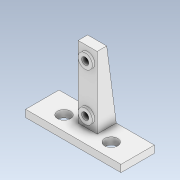
# Autodesk Inventor part: limit_switch_horizontal
Saved by Autodesk Inventor 2022 (Build 260153000, 153)
## iProperties
Created: 2022-05-08
Part Number: limit_switch_horizontal
Material: Generic
Document SubType Name: Modeling
Designer: ferna
Density: 1 g/cm^3
Appearance: White
Author: ferna
Autodesk Inventor part; units mm, degrees
ref_plane "YZ Plane" through (0, 0, 0) normal (1, 0, 0) x (0, 1, 0)
ref_plane "XZ Plane" through (0, 0, 0) normal (0, 1, 0) x (-1, 0, 0)
ref_plane "XY Plane" through (0, 0, 0) normal (0, 0, 1) x (1, 0, 0)
sketch "Sketch1" plane through (0, 0, 0) normal (0, 1, 0) x (-1, 0, 0)
  circle A0 centre (30.1, 6) radius 2.1
  circle A1 centre (49.9, 6) radius 2.1
  line L0 (0, 0) -> (80, 0)
  line L1 (80, 0) -> (80, 12)
  line L2 (0, 12) -> (80, 12)
  line L3 (0, 0) -> (0, 12)
  line L4 (40, 12) -> (15, 12)
  line L5 (15, 12) -> (15, 0)
  line L6 (15, 0) -> (65, 0)
  line L7 (65, 0) -> (65, 12)
  circle A2 centre (49.9, 6) radius 2.75
  circle A3 centre (30.1, 6) radius 2.75
  dimension "d0" = 25
  dimension "d1" = 50
  dimension "d2" = 5.5
  dimension "d3" = 5.5
  constraints: 16 end point, 4 centre point, 4 point on line, 2 coincident, 2 perpendicular, 1 midpoint
  measures "d0" distance of L4.start L4.end
  measures "d1" distance of L5.end L6.end
  measures "d2" diameter of A2
  measures "d3" diameter of A3
extrude "Extrusion1" add sketch "Sketch1" along normal blind 3 contours L5 L2 L7 L0
sketch "Sketch6" plane through (0, 3, 0) normal (0, 1, 0) x (1, 0, 0)
  line L0 (-15, 0) -> (-65, 0) projected
  line L1 (-40, 0) -> (-43, 0)
  line L2 (-65, -12) -> (-15, -12) projected
  line L3 (-40, -12) -> (-40, -8)
  line L4 (-40, -8) -> (-43, -8)
  line L5 (-43, -8) -> (-43, -4)
  line L6 (-43, -4) -> (-37, -4)
  line L7 (-37, -4) -> (-37, -8)
  line L8 (-37, -8) -> (-40, -8)
  line L9 (-43, -8) -> (-44, -8)
  line L10 (-44, -8) -> (-44, -4)
  line L11 (-44, -4) -> (-43, -4)
  line L12 (-43, -4) -> (-43, -8)
  line L13 (-37, -4) -> (-36, -4)
  line L14 (-36, -4) -> (-36, -8)
  line L15 (-36, -8) -> (-37, -8)
  line L16 (-37, -8) -> (-37, -4)
  point P0 (0, 0)
  dimension "d22" = 3
  dimension "d23" = 4
  dimension "d24" = 4
  dimension "d25" = 6
  dimension "d28" = 1
  dimension "d29" = 1
  constraints: 30 end point, 7 perpendicular, 4 parallel, 3 point on line, 2 horizontal, 2 midpoint, 1 vertical
  measures "d22" distance of L1.start L1.end
  measures "d23" distance of L3.start L3.end
  measures "d24" distance of L4.end L5.end
  measures "d25" distance of L5.end L6.end
  measures "d28" distance of L10.end L11.end
  measures "d29" distance of L14.end L15.end
extrude "Extrusion6" add sketch "Sketch6" along normal blind 30
sketch "Sketch8" plane through (-65, 0, 0) normal (-1, 0, 0) x (0, 0, 1)
  line L0 (0, 0) -> (12, 0) projected
  line L1 (12, 0) -> (12, 3) projected
  line L2 (0, 3) -> (12, 3) projected
  line L3 (0, 0) -> (0, 3) projected
extrude "Extrusion8" cut sketch "Sketch8" against normal blind 5
sketch "Sketch9" plane through (-15, 0, 12) normal (1, 0, 0) x (0, 0, -1)
  line L0 (0, 0) -> (12, 0) projected
  line L1 (12, 0) -> (12, 3) projected
  line L2 (0, 3) -> (12, 3) projected
  line L3 (0, 0) -> (0, 3) projected
extrude "Extrusion9" cut sketch "Sketch9" against normal blind 5
sketch "Sketch10" plane through (-44, 3, 4) normal (-1, 0, 0) x (0, 0, 1)
  line L0 (-4, -3) -> (-4, 0) projected
  line L1 (-4, 0) -> (0, 0)
  line L2 (-0.75, 0) -> (4.75, 0) projected
  line L3 (0, 30) -> (-4, 0)
  line L4 (0, 30) -> (4, 30) projected
  line L5 (4, 0) -> (4, 30) projected
  dimension "d41" = 4
  constraints: 4 end point, 1 point on line
  measures "d41" distance of L0.end L1.end
extrude "Extrusion10" add sketch "Sketch10" against normal blind 8
sketch "Sketch7" plane through (-36, 3, 4) normal (0, 0, -1) x (-1, 0, 0)
  line L0 (8, 0) -> (8, 30) projected
  line L1 (8, 15) -> (8, 5)
  line L2 (8, 5) -> (8, 25)
  line L3 (8, 25) -> (4, 25)
  line L4 (0, 0) -> (0, 30) projected
  line L5 (8, 5) -> (4, 5)
  circle A0 centre (4, 25) radius 1.5
  circle A1 centre (4, 5) radius 1.5
  point P0 (-36, -3)
  dimension "d30" = 10
  dimension "d31" = 20
  dimension "d32" = 4
  dimension "d33" = 3
  dimension "d34" = 3
  constraints: 8 end point, 2 centre point, 2 coincident, 2 point on line, 1 horizontal, 1 midpoint, 1 perpendicular
  measures "d30" distance of L1.start L1.end
  measures "d31" distance of L1.end L2.end
  measures "d32" distance of L2.end L3.end
  measures "d33" diameter of A0
  measures "d34" diameter of A1
extrude "Extrusion7" cut sketch "Sketch7" along normal mid plane 30
sketch "Sketch11" plane through (-44, 3, 8) normal (0, 0, 1) x (1, 0, 0)
  circle A0 centre (4, 25) radius 1.5 projected
  circle A1 centre (4, 5) radius 1.5 projected
  circle A2 centre (4, 25) radius 3
  circle A3 centre (4, 5) radius 3
  point P0 (44, -3)
  dimension "d44" = 6
  dimension "d45" = 6
  constraints: 2 centre point, 2 coincident
  measures "d44" diameter of A2
  measures "d45" diameter of A3
extrude "Extrusion11" add sketch "Sketch11" along normal blind 1
sketch "Sketch12" plane through (-60, 0, 12) normal (0, 0, 1) x (1, 0, 0)
  line L0 (40, 0) -> (40, 3) projected
  line L1 (0, 3) -> (40, 3) projected
  line L2 (0, 3) -> (0, 0) projected
  line L3 (0, 0) -> (40, 0) projected
  point P0 (60, 0)
extrude "Extrusion12" add sketch "Sketch12" along normal blind 2
sketch "Sketch13" plane through (0, 3, 0) normal (0, 1, 0) x (1, 0, 0)
  circle A0 centre (-30.1, -6) radius 2.75 projected
  circle A1 centre (-49.9, -6) radius 2.75 projected
  line L0 (-36, 0) -> (-36, -8) projected
  line L1 (-36, -8) -> (-44, -8) projected
  line L2 (-44, -8) -> (-44, 0) projected
  line L3 (-44, 0) -> (-60, 0) projected
  line L4 (-60, 0) -> (-60, -14) projected
  line L5 (-20, -14) -> (-60, -14) projected
  line L6 (-20, -14) -> (-20, 0) projected
  line L7 (-20, 0) -> (-36, 0) projected
  line L8 (-30.1, -6) -> (-30.1, -8)
  line L9 (-49.9, -6) -> (-49.9, -8)
  circle A2 centre (-49.9, -8) radius 2.75
  circle A3 centre (-30.1, -8) radius 2.75
  point P0 (0, 0)
  constraints: 4 end point, 2 centre point, 2 coincident, 2 vertical
sketch "Sketch14" plane through (0, 3, 0) normal (0, 1, 0) x (1, 0, 0)
  circle A0 centre (-49.9, -6) radius 2.75 projected
  circle A1 centre (-30.1, -6) radius 2.75 projected
  point P0 (0, 0)
extrude "Extrusion14" add sketch "Sketch13" against normal up to surface (3 mm away) contours A0 A3 | A3 A0 | A1 A2 | A2 A1 picked at (-29.7315, -4.622) picked at (-30.3176, -7.5571) picked at (-49.5315, -4.622) picked at (-50.1176, -6.4429)
sketch "Sketch15" plane through (0, 3, 0) normal (0, 1, 0) x (1, 0, 0)
  circle A0 centre (-30.1, -6) radius 2.75 projected
  circle A1 centre (-49.9, -6) radius 2.75 projected
  line L0 (-30.1, -6) -> (-30.1, -8)
  line L1 (-49.9, -6) -> (-49.9, -8)
  circle A2 centre (-49.9, -8) radius 2.75
  circle A3 centre (-30.1, -8) radius 2.75
  point P0 (0, 0)
  dimension "d54" = 2
  constraints: 4 end point, 2 centre point, 2 coincident, 2 vertical
  measures "d54" distance of L0.start L0.end
extrude "Extrusion15" cut sketch "Sketch15" against normal through all contours A3 A0 | A0 A3 | A2 A1 | A1 A2 picked at (-30.3176, -7.5571) picked at (-29.7315, -9.378) picked at (-50.1176, -6.4429) picked at (-49.5315, -9.378)
body "Solid1"
